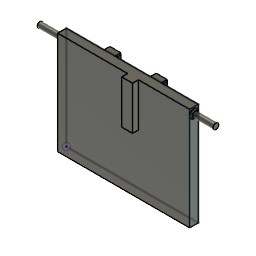
Flap01 (Autodesk Fusion 360 design; units mm, degrees)
part number: 2026-05-25-17-31-46-092
Autodesk Fusion 360 part; units mm, degrees
sketch "flap" plane through (0, 0, 0) normal (0, 1, 0) x (1, 0, 0)
  line L0 (0, 0) -> (45, 0)
  line L1 (45, 0) -> (45, -35)
  line L2 (45, -35) -> (0, -35)
  line L3 (0, -35) -> (0, 0)
  dimension "d1" = 45
  dimension "d2" = 35
  constraint coincident L0.start L3.end
  constraint horizontal L0
  constraint perpendicular L0 L1
  constraint perpendicular L1 L2
  constraint perpendicular L0 L3
  measures "d1" distance of L0.start L0.end
  measures "d2" distance of L0.end L1.end
extrude "Extrude1" add sketch "flap" against normal blind 3
sketch "prindere flap" plane through (45, 0, 0) normal (1, 0, 0) x (0, 1, 0)
  line L0 (0, 0) -> (0, 35)
  line L1 (0, 35) -> (-3, 35)
  line L2 (-3, 35) -> (-3, 0)
  line L3 (-3, 0) -> (0, 0)
  circle A0 centre (-1.5, 33) radius 1
  dimension "d20" = 2
  dimension "d21" = 2
  dimension "d22" = 1.5
  measures "d20" diameter of A0
  measures "d21" distance of L1 A0.centre
  measures "d22" distance of L2 A0.centre
extrude "Extrude4" add sketch "prindere flap" along normal blind 7.5 contours A0
extrude "Extrude5" add sketch "prindere flap" against normal blind 7.5 from surface at -45 contours A0
fillet "Fillet3" radius 0.5 2 edges at (0, -2.4323, 32.6384) (45, -2.4323, 33.3616)
sketch "Sketch8" plane through (0, 0, 0) normal (0, 1, 0) x (1, 0, 0)
  line L0 (0.6311, -53.2153) -> (44.5806, -53.2153) construction
  line L1 (44.5806, -53.2153) -> (44.5806, -19.208) construction
  line L2 (44.5806, -19.208) -> (0.6311, -19.208) construction
  line L3 (0.6311, -19.208) -> (0.6311, -53.2153) construction
  dimension "d40" = 30
  dimension "d41" = 0
  text T0 "0" font "Arial" height 30 align centre top in box 43.9494 x 34.0073 at (0.6311, -53.2153) x (1, 0) y (0, 1) spacing 1
emboss "Emboss1" depth 2 profiles "Sketch8" section 1 text T0 onto face at (15, 0, 23.3333)
sketch "Sketch9" plane through (0, -3, 0) normal (0, -1, 0) x (1, 0, 0)
  line L0 (45, 35) -> (0, 35)
  line L1 (0, 35) -> (0, 33)
  line L2 (0, 33) -> (0, 0)
  line L3 (0, 0) -> (45, 0)
  line L4 (45, 0) -> (45, 33)
  line L5 (45, 33) -> (45, 35)
  line L6 (0.5209, 17.1935) -> (43.5209, 17.1935) construction
  line L7 (43.5209, 17.1935) -> (43.5209, 50.1935) construction
  line L8 (43.5209, 50.1935) -> (0.5209, 50.1935) construction
  line L9 (0.5209, 50.1935) -> (0.5209, 17.1935) construction
  dimension "d46" = 30
  dimension "d47" = 0
  text T0 "1" font "Arial" height 30 align centre top in box 43 x 33 at (0.5209, 17.1935) x (1, 0) y (0, 1) spacing 1
emboss "Emboss2" depth 2 profiles "Sketch9" section 1 text T0 onto face at (15, -3, 23.3333)
equation "d41 = '0'"
equation "d47 = '1'"
named bodies: "flap"
